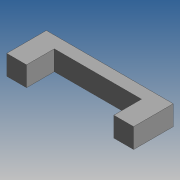
# Autodesk Inventor part: P003-Corps_piston
Saved by Autodesk Inventor 2021.4 (Build 254397000, 397)
## iProperties
Created: 2022-03-18
Part Number: P003-Corps_piston
Material: Générique
Document SubType Name: Modeling
Designer: Maintenant Prêt
Density: 1 g/cm^3
Appearance: Par défaut
Author: Maintenant Prêt
Autodesk Inventor part; units mm, degrees
ref_plane "YZ Plane" through (0, 0, 0) normal (1, 0, 0) x (0, 1, 0)
ref_plane "XZ Plane" through (0, 0, 0) normal (0, 1, 0) x (-1, 0, 0)
ref_plane "XY Plane" through (0, 0, 0) normal (0, 0, 1) x (1, 0, 0)
sketch "Sketch2" plane through (0, 0, 0) normal (0, 0, 1) x (1, 0, 0)
  line L0 (-22.4, 0) -> (22.4, 0) construction
  line L1 (0, -2) -> (0, 12) construction
  line L2 (-16, 0) -> (-16, 10)
  line L3 (-16, 10) -> (16, 10)
  line L4 (16, 10) -> (16, 0)
  line L5 (11, 0) -> (11, 7)
  line L6 (11, 7) -> (-11, 7)
  line L7 (-11, 7) -> (-11, 0)
  line L8 (-16, 0) -> (-11, 0)
  line L9 (11, 0) -> (16, 0)
  point P0 (0, 0)
  dimension "d0" = 32
  dimension "d1" = 22
  dimension "d2" = 10
  dimension "d3" = 7
  constraints: 16 end point, 4 perpendicular, 4 point on line, 2 vertical, 1 collinear, 1 horizontal, 2 other
  measures "d0" distance of L2.end L3.end
  measures "d1" distance of L5.end L6.end
  measures "d2" distance between parallel lines of L0 L3
  measures "d3" distance between parallel lines of L0 L6
extrude "Extrusion1" add sketch "Sketch2" along normal mid plane 5
body "Solid1"
